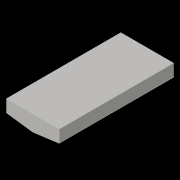
# Autodesk Inventor part: Generalcraftshape1
Saved by Autodesk Inventor 2016 (Build 200138000, 138)
## iProperties
Created: 2019-01-02
Part Number: Generalcraftshape1
Material: Generic
Document SubType Name: Modeling
Designer: LinJie
Density: 1 g/cm^3
Appearance: Default
Author: LinJie
Autodesk Inventor part; units mm, degrees
ref_plane "YZ Plane" through (0, 0, 0) normal (1, 0, 0) x (0, 1, 0)
ref_plane "XZ Plane" through (0, 0, 0) normal (0, 1, 0) x (-1, 0, 0)
ref_plane "XY Plane" through (0, 0, 0) normal (0, 0, 1) x (1, 0, 0)
sketch "Sketch1" plane through (0, 0, 0) normal (0, 1, 0) x (-1, 0, 0)
  line L0 (15, 7) -> (-15, 7)
  line L1 (-15, 7) -> (-15, 0)
  line L2 (-15, 0) -> (15, 0)
  line L3 (15, 0) -> (15, 7)
  line L4 (15, 0) -> (0, -2)
  line L5 (0, -2) -> (-15, 0)
  point P0 (0, 0)
  point P1 (0, 0)
  dimension "d0" = 30
  dimension "d1" = 7
  dimension "d2" = 2
  constraints: 12 end point, 2 parallel, 1 coincident, 1 equal length, 1 horizontal, 1 midpoint, 1 perpendicular
  measures "d0" distance of L1.end L2.end
  measures "d1" distance of L0.end L1.end
  measures "d2" distance of L4.end point (0, 0)
extrude "Extrusion1" add sketch "Sketch1" along normal blind 65
body "Solid1"
